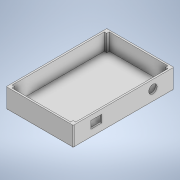
# Autodesk Inventor part: señales_carcasa_x10
Saved by Autodesk Inventor 2022 (Build 260153000, 153)
## iProperties
Created: 2023-06-20
Part Number: señales_carcasa_x10
Material: Generic
Document SubType Name: Modeling
Designer: Asus
Density: 1 g/cm^3
Appearance: Default
Author: Asus
Autodesk Inventor part; units mm, degrees
ref_plane "YZ Plane" through (0, 0, 0) normal (1, 0, 0) x (0, 1, 0)
ref_plane "XZ Plane" through (0, 0, 0) normal (0, 1, 0) x (-1, 0, 0)
ref_plane "XY Plane" through (0, 0, 0) normal (0, 0, 1) x (1, 0, 0)
sketch "Sketch1" plane through (0, 0, 0) normal (0, 1, 0) x (-1, 0, 0)
  line L0 (-400, 600) -> (400, 600)
  line L1 (400, 600) -> (400, -600)
  line L2 (400, -600) -> (-400, -600)
  line L3 (-400, -600) -> (-400, 600)
  line L4 (-400, 600) -> (400, -600) construction
  line L5 (400, 600) -> (-400, -600) construction
  point P0 (0, 0)
  dimension "d0" = 800
  dimension "d1" = 1200
  constraints: 12 end point, 2 midpoint, 2 parallel, 1 horizontal, 1 perpendicular
  measures "d0" distance of L1.end L2.end
  measures "d1" distance of L0.end L1.end
extrude "Extrusion1" add sketch "Sketch1" along normal blind 235
sketch "Sketch2" plane through (0, 0, 0) normal (0, -1, 0) x (1, 0, 0)
  line L0 (200, 400) -> (-200, 400)
  line L1 (-200, 400) -> (-200, 420)
  line L2 (-200, 420) -> (200, 420)
  line L3 (200, 420) -> (200, 400)
  line L4 (200, 400) -> (-200, 420) construction
  line L5 (-200, 400) -> (200, 420) construction
  line L6 (200, -420) -> (-200, -420)
  line L7 (-200, -420) -> (-200, -400)
  line L8 (-200, -400) -> (200, -400)
  line L9 (200, -400) -> (200, -420)
  line L10 (200, -420) -> (-200, -400) construction
  line L11 (-200, -420) -> (200, -400) construction
  line L12 (400, -600) -> (-400, -600) projected
  line L13 (400, 600) -> (400, -600) projected
  point P0 (0, 0)
  point P1 (0, 410)
  point P2 (0, -410)
  dimension "d4" = 400
  dimension "d5" = 20
  dimension "d6" = 400
  dimension "d7" = 20
  dimension "d9" = 800
  dimension "d10" = 180
  dimension "d11" = 200
  dimension "d12" = 200
  constraints: 24 end point, 5 parallel, 4 midpoint, 2 horizontal, 2 perpendicular
  measures "d4" distance of L1.end L2.end
  measures "d5" distance of L0.end L1.end
  measures "d6" distance of L7.end L8.end
  measures "d7" distance of L6.end L7.end
  measures "d9" distance between parallel lines of L0 L8
  measures "d10" distance between parallel lines of L12 L6
  measures "d11" distance between parallel lines of L13 L9
  measures "d12" distance between parallel lines of L13 L3
extrude "Extrusion2" add sketch "Sketch2" along normal blind 35
sketch "Sketch3" plane through (-200, 0, 420) normal (0, 0, 1) x (1, 0, 0)
  line L0 (10, -10) -> (390, -10)
  line L1 (390, -10) -> (390, -25)
  line L2 (390, -25) -> (10, -25)
  line L3 (10, -25) -> (10, -10)
  line L4 (10, -10) -> (390, -25) construction
  line L5 (390, -10) -> (10, -25) construction
  line L6 (400, -35) -> (0, -35) projected
  line L7 (400, 0) -> (400, -35) projected
  point P0 (200, 0)
  point P1 (200, -17.5)
  dimension "d15" = 380
  dimension "d16" = 15
  dimension "d17" = 10
  dimension "d18" = 10
  constraints: 12 end point, 2 midpoint, 2 parallel, 1 horizontal, 1 perpendicular
  measures "d15" distance of L1.end L2.end
  measures "d16" distance of L0.end L1.end
  measures "d17" distance between parallel lines of L6 L2
  measures "d18" distance between parallel lines of L7 L1
extrude "Extrusion3" cut sketch "Sketch3" against normal blind 1000
fillet "Fillet1" radius 10 8 edges at (0, 0, 600) (400, 0, 0) (400, 117.5, 600) (-400, 117.5, 600) (-400, 0, 0) (-400, 117.5, -600) (0, 0, -600) (400, 117.5, -600)
sketch "Sketch8" plane through (400, 10, 590) normal (1, 0, 0) x (0, 0, -1)
  line L0 (940, 225) -> (940, 25) construction
  circle A0 centre (940, 125) radius 50
  line L1 (0, 225) -> (1180, 225) projected
  line L2 (0, -10) -> (1180, -10) projected
  line L3 (1190, 0) -> (1190, 225) projected
  line L4 (200, 80) -> (330, 80)
  line L5 (330, 80) -> (330, 170)
  line L6 (330, 170) -> (200, 170)
  line L7 (200, 170) -> (200, 80)
  line L8 (200, 80) -> (330, 170) construction
  line L9 (330, 80) -> (200, 170) construction
  line L10 (940, 125) -> (0, 125) construction
  line L11 (0, 0) -> (0, 225) projected
  point P0 (590, -10)
  point P1 (265, 125)
  point P2 (265, 125)
  dimension "d39" = 100
  dimension "d40" = 35
  dimension "d41" = 250
  dimension "d44" = 130
  dimension "d45" = 90
  dimension "d46" = 200
  constraints: 16 end point, 4 midpoint, 3 point on line, 2 horizontal, 2 parallel, 2 perpendicular, 1 centre point
  measures "d39" diameter of A0
  measures "d40" distance from line of L2 L0.end
  measures "d41" distance between parallel lines of L3 L0
  measures "d44" distance of L6.end L5.end
  measures "d45" distance of L5.end L4.end
  measures "d46" distance between parallel lines of L7 L11
extrude "Extrusion7" cut sketch "Sketch8" against normal blind 50
sketch "Sketch9" plane through (0, 235, 0) normal (0, 1, 0) x (1, 0, 0)
  line L0 (-380, -550) -> (380, -550)
  line L1 (380, -550) -> (380, 550)
  line L2 (380, 550) -> (-380, 550)
  line L3 (-380, 550) -> (-380, -550)
  line L4 (-380, -550) -> (380, 550) construction
  line L5 (380, -550) -> (-380, 550) construction
  line L6 (400, -590) -> (400, 590) projected
  line L7 (390, 600) -> (-390, 600) projected
  line L8 (-350, -580) -> (350, -580)
  line L9 (350, -580) -> (350, 580)
  line L10 (350, 580) -> (-350, 580)
  line L11 (-350, 580) -> (-350, -580)
  line L12 (-350, -580) -> (350, 580) construction
  line L13 (350, -580) -> (-350, 580) construction
  point P0 (0, 0)
  point P1 (-350, -550)
  point P2 (350, -550)
  point P3 (350, 550)
  point P4 (-350, 550)
  dimension "d47" = 20
  dimension "d48" = 50
  dimension "d49" = 50
  dimension "d50" = 20
  constraints: 24 end point, 4 midpoint, 4 parallel, 2 horizontal, 2 perpendicular
  measures "d47" distance between parallel lines of L6 L1
  measures "d48" distance between parallel lines of L7 L2
  measures "d49" distance between parallel lines of L6 L9
  measures "d50" distance between parallel lines of L7 L10
extrude "Extrusion8" cut sketch "Sketch9" against normal blind 200
body "Solid1"
